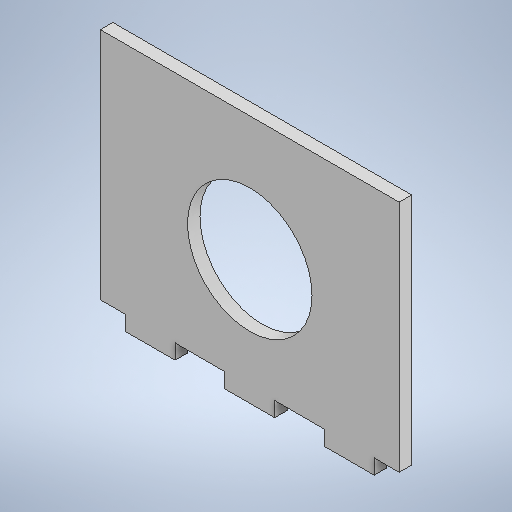
# Autodesk Inventor part: Archimedes Screw Border1
Saved by Autodesk Inventor 2025.3 (Build 293356000, 356)
## iProperties
Created: 2026-03-14
Part Number: Archimedes Screw Border1
Material: Generic
Document SubType Name: Modeling
Designer: ziada
Density: 1 g/cm^3
Appearance: Default
Author: ziada
Autodesk Inventor part; units mm, degrees
ref_plane "YZ Plane" through (0, 0, 0) normal (1, 0, 0) x (0, 1, 0)
ref_plane "XZ Plane" through (0, 0, 0) normal (0, 1, 0) x (-1, 0, 0)
ref_plane "XY Plane" through (0, 0, 0) normal (0, 0, 1) x (1, 0, 0)
sketch "Sketch1" plane through (0, 0, 0) normal (0, 0, 1) x (1, 0, 0)
  line L0 (0, 0) -> (0, 100)
  line L1 (0, 100) -> (120, 100)
  line L2 (120, 100) -> (120, 0)
  line L3 (120, 0) -> (0, 0)
  circle A0 centre (60, 50) radius 25
  line L4 (0, 0) -> (0, 6)
  line L5 (0, 6) -> (10, 6)
  line L6 (10, 6) -> (10, 0)
  line L7 (10, 0) -> (30, 0)
  line L8 (30, 0) -> (30, 6)
  line L9 (30, 6) -> (50, 6)
  line L10 (50, 6) -> (50, 0)
  line L11 (50, 0) -> (70, 0)
  line L12 (70, 0) -> (70, 6)
  line L13 (70, 6) -> (90, 6)
  line L14 (90, 6) -> (90, 0)
  line L15 (90, 0) -> (110, 0)
  line L16 (110, 0) -> (110, 6)
  line L17 (110, 6) -> (120, 6)
  dimension "d3" = 100
  dimension "d4" = 120
  dimension "d6" = 50
  dimension "d9" = 50
  dimension "d10" = 60
  dimension "d11" = 6
  dimension "d12" = 10
  dimension "d13" = 20
  dimension "d14" = 20
  dimension "d15" = 20
  dimension "d16" = 20
  dimension "d17" = 20
  constraints: 36 end point, 12 point on line, 9 perpendicular, 3 parallel, 1 centre point, 1 vertical
  measures "d3" distance of L0.start L0.end
  measures "d4" distance of L0.end L1.end
  measures "d6" diameter of A0
  measures "d9" distance from line of L3 A0.centre
  measures "d10" distance from line of L0 A0.centre
  measures "d11" distance of L0.start L4.end
  measures "d12" distance of L4.end L5.end
  measures "d13" distance of L6.end L7.end
  measures "d14" distance of L8.end L9.end
  measures "d15" distance of L10.end L11.end
  measures "d16" distance of L12.end L13.end
  measures "d17" distance of L14.end L15.end
extrude "Extrusion1" add sketch "Sketch1" against normal blind 5 contours L0 L1 L2 L17 L16 L3 L14 L13 L12 L10 L9 L8 L6 L5
body "Solid1"
